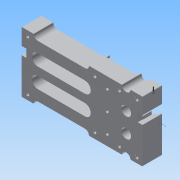
# Autodesk Inventor part: Core_bottom-im
Saved by Autodesk Inventor 2016 (Build 200138000, 138)
## iProperties
Created: 2015-05-18
Part Number: Core_bottom-im
Material: ABS Plastic
Document SubType Name: Modeling
Designer: Openlab
Density: 1.06 g/cm^3
Appearance: Smooth - White
Mass: 36.0444 g
Surface Area: 283.752 cm^2
Volume: 34.0041 cm^3
Author: Openlab
Autodesk Inventor part; units mm, degrees
ref_plane "YZ Plane" through (0, 0, 0) normal (1, 0, 0) x (0, 1, 0)
ref_plane "XZ Plane" through (0, 0, 0) normal (0, 1, 0) x (-1, 0, 0)
ref_plane "XY Plane" through (0, 0, 0) normal (0, 0, 1) x (1, 0, 0)
sketch "Sketch1" plane through (0, 0, 0) normal (0, 1, 0) x (-1, 0, 0)
  line L0 (6.75, 23.75) -> (-6.75, 23.75)
  line L1 (-6.75, 23.75) -> (-6.75, 19.5)
  line L2 (-6.75, 10.25) -> (6.75, 10.25)
  line L3 (6.75, 10.25) -> (6.75, 14.5)
  line L4 (56.9183, 17) -> (21.35, 17) construction
  line L5 (69.8, -24.75) -> (69.8, -20.1)
  line L6 (-26.8, 24.75) -> (-26.8, 12.5)
  line L7 (9.25, 15) -> (7.25, 15)
  line L8 (7.25, 19) -> (9.25, 19)
  line L9 (-7.25, 15) -> (-9.25, 15)
  line L10 (-9.25, 19) -> (-7.25, 19)
  line L11 (-12.05, 19) -> (-24.5, 19)
  line L12 (-12.05, 15) -> (-24.5, 15)
  line L13 (21.8266, 8.5) -> (74, 8.5) construction
  line L14 (67.5, 20.5) -> (66, 20.5)
  line L15 (66, 13.5) -> (67.5, 13.5)
  line L16 (-31, 4.5) -> (-31, -25.75)
  line L17 (21.35, -8.5) -> (74, -8.5) construction
  line L18 (6.75, 6.75) -> (-6.75, 6.75)
  line L19 (-6.75, 6.75) -> (-6.75, 2.5)
  line L20 (-6.75, -6.75) -> (6.75, -6.75)
  line L21 (6.75, -6.75) -> (6.75, -2.5)
  line L22 (56.8064, 0) -> (19.3437, 0) construction
  line L23 (0, 20.1335) -> (0, -26.25) construction
  line L24 (9.25, -2) -> (7.25, -2)
  line L25 (7.25, 2) -> (9.25, 2)
  line L26 (67.5, 3.5) -> (66, 3.5)
  line L27 (66, -3.5) -> (67.5, -3.5)
  line L28 (6.75, -10.25) -> (-6.75, -10.25)
  line L29 (6.75, -23.75) -> (6.75, -19.5)
  line L30 (-6.75, -23.75) -> (6.75, -23.75)
  line L31 (55.9522, -17) -> (21.0014, -17) construction
  line L32 (67.5, -13.5) -> (66, -13.5)
  line L33 (66, -20.5) -> (67.5, -20.5)
  line L34 (9.25, -19) -> (7.25, -19)
  line L35 (73.5, 5) -> (72.5, 5)
  line L36 (70.3, 12) -> (72.5, 12)
  line L37 (-9.25, -15) -> (-7.25, -15)
  line L38 (-7.25, -19) -> (-9.25, -19)
  line L39 (-12.05, -19) -> (-24.5, -19)
  line L40 (-9.25, 2) -> (-7.25, 2)
  line L41 (-7.25, -2) -> (-9.25, -2)
  line L42 (-12.05, -2) -> (-24.5, -2)
  line L43 (-29.5, 5) -> (-30.5, 5)
  line L44 (-30.5, 12) -> (-29.5, 12)
  line L45 (67.5, 5.5) -> (66, 5.5)
  line L46 (66, 5.5) -> (66, 11.5)
  line L47 (66, 11.5) -> (67.5, 11.5)
  line L48 (-24.5, 5.5) -> (-23, 5.5)
  line L49 (-23, 5.5) -> (-23, 11.5)
  line L50 (-23, 11.5) -> (-24.5, 11.5)
  line L51 (-25, 24.75) -> (-25, 19.5)
  line L52 (-25, 5) -> (-25, 2.5)
  arc A0 (18.9998, 13.5) -> (19, 3.5) centre (19, 8.5) ccw
  arc A1 (60, 3.5) -> (60, 13.5) centre (60, 8.5) ccw
  arc A2 (19, -3.5) -> (19, -13.5) centre (19, -8.5) ccw
  arc A3 (60, -13.5) -> (60, -3.5) centre (60, -8.5) ccw
  line L53 (18.9998, 13.5) -> (60, 13.5)
  line L54 (19, 3.5) -> (60, 3.5)
  line L55 (19, -3.5) -> (60, -3.5)
  line L56 (19, -13.5) -> (60, -13.5)
  arc A4 (-16.55, -12.5) -> (-16.55, -4.5) centre (-16.55, -8.5) ccw
  line L57 (72.5, -24.75) -> (72.5, -19.6)
  line L58 (-29.5, 24.75) -> (-29.5, 12)
  arc A5 (-17, -4.5) -> (-17, -12.5) centre (-17, -8.5) ccw
  arc A6 (-17, 12.5) -> (-17, 4.5) centre (-17, 8.5) ccw
  line L59 (-16.55, -12.5) -> (-17, -12.5)
  line L60 (-17, -4.5) -> (-16.55, -4.5)
  line L61 (-17, 4.5) -> (-16.55, 4.5)
  line L62 (-16.55, 12.5) -> (-17, 12.5)
  arc A7 (-16.55, 4.5) -> (-16.55, 12.5) centre (-16.55, 8.5) ccw
  line L63 (59.3387, -15) -> (12.05, -15)
  line L64 (59.3387, -19) -> (12.05, -19)
  line L65 (59.3387, -2) -> (12.05, -2)
  line L66 (59.3387, 2) -> (12.05, 2)
  line L67 (59.3387, 15) -> (12.05, 15)
  line L68 (59.3387, 19) -> (12.05, 19)
  arc A8 (61, -14.4) -> (59.3387, -15) centre (61, -17) ccw
  arc A9 (59.3387, -19) -> (61, -19.6) centre (61, -17) ccw
  arc A10 (61, 2.6) -> (59.3387, 2) centre (61, 0) ccw
  arc A11 (59.3387, -2) -> (61, -2.6) centre (61, 0) ccw
  arc A12 (61, 19.6) -> (59.3387, 19) centre (61, 17) ccw
  arc A13 (59.3387, 15) -> (61, 14.4) centre (61, 17) ccw
  arc A14 (63.4725, -25.8125) -> (60, -22.75) centre (60, -26.25) ccw
  arc A15 (19, -22.75) -> (15.5275, -25.8125) centre (19, -26.25) ccw
  arc A16 (64.7697, -24.75) -> (60, -21.25) centre (60, -26.25) ccw
  line L69 (60, -21.25) -> (18.9998, -21.25)
  line L70 (63.9686, -26.25) -> (73.5, -26.25)
  line L71 (60, -22.75) -> (19, -22.75)
  arc A17 (18.9998, -21.25) -> (14.2303, -24.75) centre (19, -26.25) ccw
  arc A18 (14.2559, 24.6709) -> (18.9998, 21.25) centre (19, 26.25) ccw
  arc A19 (15.5275, 25.8125) -> (19, 22.75) centre (19, 26.25) ccw
  line L72 (60, 22.75) -> (19, 22.75)
  line L73 (60, 21.25) -> (18.9998, 21.25)
  line L74 (64.7697, 24.75) -> (69.8, 24.75)
  line L75 (73.5, 26.25) -> (63.9686, 26.25)
  arc A20 (60, 22.75) -> (63.4725, 25.8125) centre (60, 26.25) ccw
  arc A21 (60, 21.25) -> (64.7697, 24.75) centre (60, 26.25) ccw
  arc A22 (-13.0775, -25.8125) -> (-16.55, -22.75) centre (-16.55, -26.25) ccw
  arc A23 (-17, -22.75) -> (-20.4725, -25.8125) centre (-17, -26.25) ccw
  line L76 (-16.55, -21.25) -> (-17, -21.25)
  line L77 (-16.55, -22.75) -> (-17, -22.75)
  arc A24 (-17, -21.25) -> (-21.7697, -24.75) centre (-17, -26.25) ccw
  arc A25 (-11.7803, -24.75) -> (-16.55, -21.25) centre (-16.55, -26.25) ccw
  line L78 (14.2303, -24.75) -> (-11.7803, -24.75)
  line L79 (-21.7697, -24.75) -> (-29.5, -24.75)
  line L80 (-30.5, -26.25) -> (-20.9686, -26.25)
  line L81 (14.7303, -26.25) -> (15.0314, -26.25)
  line L82 (-16.55, 21.25) -> (-17, 21.25)
  line L83 (-16.55, 22.75) -> (-17, 22.75)
  arc A26 (-20.4725, 25.8125) -> (-17, 22.75) centre (-17, 26.25) ccw
  arc A27 (-16.55, 22.75) -> (-13.0775, 25.8125) centre (-16.55, 26.25) ccw
  arc A28 (-21.7697, 24.75) -> (-17, 21.25) centre (-17, 26.25) ccw
  arc A29 (-16.55, 21.25) -> (-11.836, 24.5833) centre (-16.55, 26.25) ccw
  line L84 (15.0314, 26.25) -> (14.7303, 26.25)
  line L85 (-20.9686, 26.25) -> (-30.5, 26.25)
  line L86 (-29.5, 24.75) -> (-21.7697, 24.75)
  line L87 (-11.8074, 24.75) -> (14.2303, 24.75)
  line L88 (14.2303, -24.75) -> (14.2303, -25.75)
  line L89 (-11.7803, -24.75) -> (-11.7803, -25.75)
  line L90 (-11.8074, 24.75) -> (-11.8074, 25.75)
  line L91 (14.2303, 24.8288) -> (14.2303, 25.75)
  line L92 (72.5, 12) -> (73.5, 12)
  line L93 (72.5, 5) -> (70.3, 5)
  line L94 (-27.3, 12) -> (-29.5, 12)
  line L95 (-27.3, 5) -> (-29.5, 5)
  line L96 (11.55, -21) -> (9.75, -21)
  line L97 (9.75, 21) -> (11.55, 21)
  line L98 (-9.75, -21) -> (-11.55, -21)
  line L99 (-11.55, 21) -> (-9.75, 21)
  line L100 (11.55, -2.5) -> (11.55, -14.5)
  line L101 (11.55, -19.5) -> (11.55, -21)
  line L102 (9.75, -21) -> (9.75, -19.5)
  line L103 (11.55, 21) -> (11.55, 19.5)
  line L104 (11.55, 14.5) -> (11.55, 2.5)
  line L105 (9.75, 2.5) -> (9.75, 14.5)
  line L106 (9.75, 19.5) -> (9.75, 21)
  line L107 (-9.75, -2.5) -> (-9.75, -14.5)
  line L108 (-9.75, -19.5) -> (-9.75, -21)
  line L109 (-11.55, -21) -> (-11.55, -19.5)
  line L110 (-11.55, -14.5) -> (-11.55, -2.5)
  line L111 (-9.75, 21) -> (-9.75, 19.5)
  line L112 (-9.75, 14.5) -> (-9.75, 2.5)
  line L113 (-11.55, 2.5) -> (-11.55, 14.5)
  line L114 (-11.55, 19.5) -> (-11.55, 21)
  line L115 (67.5, -11.5) -> (66, -11.5)
  line L116 (66, -11.5) -> (66, -5.5)
  line L117 (66, -5.5) -> (67.5, -5.5)
  line L118 (68, -21) -> (68, -24.75)
  arc A30 (9.75, -19.5) -> (9.25, -19) centre (9.25, -19.5) ccw
  arc A31 (12.05, -19) -> (11.55, -19.5) centre (12.05, -19.5) ccw
  arc A32 (9.75, -2.5) -> (9.25, -2) centre (9.25, -2.5) ccw
  arc A33 (12.05, -2) -> (11.55, -2.5) centre (12.05, -2.5) ccw
  arc A34 (11.55, 2.5) -> (12.05, 2) centre (12.05, 2.5) ccw
  arc A35 (9.25, 2) -> (9.75, 2.5) centre (9.25, 2.5) ccw
  arc A36 (9.75, 14.5) -> (9.25, 15) centre (9.25, 14.5) ccw
  arc A37 (12.05, 15) -> (11.55, 14.5) centre (12.05, 14.5) ccw
  arc A38 (11.55, 19.5) -> (12.05, 19) centre (12.05, 19.5) ccw
  arc A39 (9.25, 19) -> (9.75, 19.5) centre (9.25, 19.5) ccw
  arc A40 (-9.75, 19.5) -> (-9.25, 19) centre (-9.25, 19.5) ccw
  arc A41 (-12.05, 19) -> (-11.55, 19.5) centre (-12.05, 19.5) ccw
  arc A42 (-11.55, 14.5) -> (-12.05, 15) centre (-12.05, 14.5) ccw
  arc A43 (-9.25, 15) -> (-9.75, 14.5) centre (-9.25, 14.5) ccw
  arc A44 (-9.75, 2.5) -> (-9.25, 2) centre (-9.25, 2.5) ccw
  arc A45 (-12.05, 2) -> (-11.55, 2.5) centre (-12.05, 2.5) ccw
  arc A46 (-11.55, -2.5) -> (-12.05, -2) centre (-12.05, -2.5) ccw
  arc A47 (-9.25, -2) -> (-9.75, -2.5) centre (-9.25, -2.5) ccw
  arc A48 (-9.75, -14.5) -> (-9.25, -15) centre (-9.25, -14.5) ccw
  arc A49 (-12.05, -15) -> (-11.55, -14.5) centre (-12.05, -14.5) ccw
  arc A50 (-9.25, -19) -> (-9.75, -19.5) centre (-9.25, -19.5) ccw
  arc A51 (-11.55, -19.5) -> (-12.05, -19) centre (-12.05, -19.5) ccw
  line L119 (65.5, -19.6) -> (61, -19.6)
  line L120 (66, -13.5) -> (66, -13.9)
  line L121 (61, -14.4) -> (65.5, -14.4)
  line L122 (65.5, -2.6) -> (61, -2.6)
  line L123 (66, 3.5) -> (66, 3.1)
  line L124 (66, -3.1) -> (66, -3.5)
  line L125 (61, 2.6) -> (65.5, 2.6)
  line L126 (65.5, 14.4) -> (61, 14.4)
  line L127 (66, 20.5) -> (66, 20.1)
  line L128 (66, 13.9) -> (66, 13.5)
  line L129 (61, 19.6) -> (65.5, 19.6)
  arc A52 (65.5, -14.4) -> (66, -13.9) centre (65.5, -13.9) ccw
  arc A53 (68, -12) -> (67.5, -11.5) centre (67.5, -12) ccw
  arc A54 (67.5, -5.5) -> (68, -5) centre (67.5, -5) ccw
  arc A55 (68, 5) -> (67.5, 5.5) centre (67.5, 5) ccw
  arc A56 (67.5, 11.5) -> (68, 12) centre (67.5, 12) ccw
  arc A57 (66, -3.1) -> (65.5, -2.6) centre (65.5, -3.1) ccw
  arc A58 (65.5, 2.6) -> (66, 3.1) centre (65.5, 3.1) ccw
  arc A59 (66, 13.9) -> (65.5, 14.4) centre (65.5, 13.9) ccw
  arc A60 (65.5, 19.6) -> (66, 20.1) centre (65.5, 20.1) ccw
  line L130 (72.5, -2.6) -> (72.5, 2.6)
  line L131 (72.5, -2.6) -> (70.3, -2.6)
  line L132 (66, -20.5) -> (66, -20.1)
  arc A61 (66, -20.1) -> (65.5, -19.6) centre (65.5, -20.1) ccw
  line L133 (68, -13) -> (68, -12)
  line L134 (68, 4) -> (68, 5)
  line L135 (68, 21) -> (68, 24.75)
  line L136 (72.5, -19.6) -> (72.5, -14.4)
  line L137 (72.5, -19.6) -> (70.3, -19.6)
  line L138 (72.5, -24.75) -> (69.8, -24.75)
  line L139 (69.8, -24.75) -> (68, -24.75)
  line L140 (68, -24.75) -> (64.7697, -24.75)
  line L141 (70.3, -14.4) -> (72.5, -14.4)
  line L142 (72.5, -14.4) -> (72.5, -2.6)
  line L143 (69.8, -13.9) -> (69.8, -3.1)
  line L144 (68, -4) -> (68, -5)
  line L145 (72.5, 2.6) -> (72.5, 5)
  line L146 (70.3, 2.6) -> (72.5, 2.6)
  line L147 (69.8, 3.1) -> (69.8, 4.5)
  line L148 (72.5, 14.4) -> (72.5, 19.6)
  line L149 (72.5, 14.4) -> (70.3, 14.4)
  line L150 (74, -25.75) -> (74, 4.5)
  line L151 (72.5, 19.6) -> (72.5, 24.75)
  line L152 (69.8, 20.1) -> (69.8, 24.75)
  line L153 (70.3, 19.6) -> (72.5, 19.6)
  line L154 (72.5, 12) -> (72.5, 14.4)
  line L155 (69.8, 24.75) -> (72.5, 24.75)
  line L156 (69.8, 12.5) -> (69.8, 13.9)
  line L157 (68, 13) -> (68, 12)
  arc A62 (67.5, -13.5) -> (68, -13) centre (67.5, -13) ccw
  arc A63 (68, -4) -> (67.5, -3.5) centre (67.5, -4) ccw
  arc A64 (67.5, 3.5) -> (68, 4) centre (67.5, 4) ccw
  arc A65 (68, 13) -> (67.5, 13.5) centre (67.5, 13) ccw
  arc A66 (67.5, 20.5) -> (68, 21) centre (67.5, 21) ccw
  arc A67 (70.3, -19.6) -> (69.8, -20.1) centre (70.3, -20.1) ccw
  arc A68 (69.8, -13.9) -> (70.3, -14.4) centre (70.3, -13.9) ccw
  arc A69 (70.3, -2.6) -> (69.8, -3.1) centre (70.3, -3.1) ccw
  arc A70 (69.8, 3.1) -> (70.3, 2.6) centre (70.3, 3.1) ccw
  arc A71 (70.3, 14.4) -> (69.8, 13.9) centre (70.3, 13.9) ccw
  arc A72 (69.8, 20.1) -> (70.3, 19.6) centre (70.3, 20.1) ccw
  line L158 (69.8, 5) -> (69.8, 12)
  line L159 (-25, 14.5) -> (-25, 12)
  line L160 (-25, -2.5) -> (-25, -14.5)
  line L161 (-25, -19.5) -> (-25, -24.75)
  line L162 (-29.5, 5) -> (-29.5, -24.75)
  arc A73 (-25, 12) -> (-24.5, 11.5) centre (-24.5, 12) ccw
  arc A74 (-24.5, 5.5) -> (-25, 5) centre (-24.5, 5) ccw
  arc A75 (68, -21) -> (67.5, -20.5) centre (67.5, -21) ccw
  arc A76 (70.3, 5) -> (69.8, 4.5) centre (70.3, 4.5) ccw
  arc A77 (69.8, 12.5) -> (70.3, 12) centre (70.3, 12.5) ccw
  line L163 (69.8, 5) -> (70.3, 5)
  line L164 (69.8, 12) -> (70.3, 12)
  arc A78 (74, 4.5) -> (73.5, 5) centre (73.5, 4.5) ccw
  line L165 (74, 25.75) -> (74, 12.5)
  arc A79 (73.5, 12) -> (74, 12.5) centre (73.5, 12.5) ccw
  line L166 (74, 4.5) -> (74, 12.5)
  arc A80 (-30.5, 5) -> (-31, 4.5) centre (-30.5, 4.5) ccw
  line L167 (-31, 12.5) -> (-31, 25.75)
  arc A81 (-31, 12.5) -> (-30.5, 12) centre (-30.5, 12.5) ccw
  line L168 (-31, 4.5) -> (-31, 12.5)
  line L169 (-26.8, -24.75) -> (-26.8, 4.5)
  arc A82 (-27.3, 12) -> (-26.8, 12.5) centre (-27.3, 12.5) ccw
  arc A83 (-26.8, 4.5) -> (-27.3, 5) centre (-27.3, 4.5) ccw
  line L170 (-26.8, 5) -> (-26.8, 12)
  line L171 (-27.3, 12) -> (-26.8, 12)
  line L172 (-27.3, 5) -> (-26.8, 5)
  arc A84 (73.5, -26.25) -> (74, -25.75) centre (73.5, -25.75) ccw
  arc A85 (63.4725, -25.8125) -> (63.9686, -26.25) centre (63.9686, -25.75) ccw
  arc A86 (15.0314, -26.25) -> (15.5275, -25.8125) centre (15.0314, -25.75) ccw
  arc A87 (-13.0775, -25.8125) -> (-12.5814, -26.25) centre (-12.5814, -25.75) ccw
  arc A88 (-20.9686, -26.25) -> (-20.4725, -25.8125) centre (-20.9686, -25.75) ccw
  arc A89 (-31, -25.75) -> (-30.5, -26.25) centre (-30.5, -25.75) ccw
  arc A90 (-30.5, 26.25) -> (-31, 25.75) centre (-30.5, 25.75) ccw
  arc A91 (-20.4725, 25.8125) -> (-20.9686, 26.25) centre (-20.9686, 25.75) ccw
  arc A92 (-12.5814, 26.25) -> (-13.0775, 25.8125) centre (-12.5814, 25.75) ccw
  arc A93 (15.5275, 25.8125) -> (15.0314, 26.25) centre (15.0314, 25.75) ccw
  arc A94 (63.9686, 26.25) -> (63.4725, 25.8125) centre (63.9686, 25.75) ccw
  arc A95 (74, 25.75) -> (73.5, 26.25) centre (73.5, 25.75) ccw
  line L173 (6.75, -19.5) -> (6.75, -14.5)
  line L174 (6.75, -14.5) -> (6.75, -10.25)
  line L175 (-6.75, -14.5) -> (-6.75, -19.5)
  line L176 (-6.75, -19.5) -> (-6.75, -23.75)
  arc A96 (7.25, -19) -> (6.75, -19.5) centre (7.25, -19.5) ccw
  arc A97 (6.75, -14.5) -> (7.25, -15) centre (7.25, -14.5) ccw
  arc A98 (-6.75, -19.5) -> (-7.25, -19) centre (-7.25, -19.5) ccw
  arc A99 (11.55, -14.5) -> (12.05, -15) centre (12.05, -14.5) ccw
  line L177 (9.75, -2.5) -> (9.75, -14.5)
  line L178 (9.25, -15) -> (7.25, -15)
  arc A100 (9.25, -15) -> (9.75, -14.5) centre (9.25, -14.5) ccw
  line L179 (-6.75, -10.25) -> (-6.75, -14.5)
  arc A101 (-7.25, -15) -> (-6.75, -14.5) centre (-7.25, -14.5) ccw
  line L180 (6.75, -2.5) -> (6.75, 2.5)
  line L181 (6.75, 2.5) -> (6.75, 6.75)
  line L182 (-6.75, -2.5) -> (-6.75, -6.75)
  line L183 (-6.75, 2.5) -> (-6.75, -2.5)
  line L184 (6.75, 14.5) -> (6.75, 19.5)
  line L185 (6.75, 19.5) -> (6.75, 23.75)
  line L186 (-6.75, 19.5) -> (-6.75, 14.5)
  line L187 (-6.75, 14.5) -> (-6.75, 10.25)
  arc A102 (7.25, -2) -> (6.75, -2.5) centre (7.25, -2.5) ccw
  arc A103 (6.75, 2.5) -> (7.25, 2) centre (7.25, 2.5) ccw
  arc A104 (-6.75, -2.5) -> (-7.25, -2) centre (-7.25, -2.5) ccw
  arc A105 (-7.25, 2) -> (-6.75, 2.5) centre (-7.25, 2.5) ccw
  arc A106 (7.25, 15) -> (6.75, 14.5) centre (7.25, 14.5) ccw
  arc A107 (6.75, 19.5) -> (7.25, 19) centre (7.25, 19.5) ccw
  arc A108 (-7.25, 19) -> (-6.75, 19.5) centre (-7.25, 19.5) ccw
  arc A109 (-6.75, 14.5) -> (-7.25, 15) centre (-7.25, 14.5) ccw
  arc A110 (14.2303, -25.75) -> (14.7303, -26.25) centre (14.7303, -25.75) ccw
  line L188 (-12.5814, -26.25) -> (-12.2803, -26.25)
  line L189 (-12.2803, -26.25) -> (14.7303, -26.25)
  arc A111 (-12.2803, -26.25) -> (-11.7803, -25.75) centre (-12.2803, -25.75) ccw
  arc A112 (14.7303, 26.25) -> (14.2303, 25.75) centre (14.7303, 25.75) ccw
  line L190 (-12.5814, 26.25) -> (-12.3074, 26.25)
  line L191 (-12.3074, 26.25) -> (14.7303, 26.25)
  arc A113 (-11.8074, 25.75) -> (-12.3074, 26.25) centre (-12.3074, 25.75) ccw
  arc A114 (14.2303, 24.8288) -> (14.2559, 24.6709) centre (14.7303, 24.8288) ccw
  arc A115 (-11.836, 24.5833) -> (-11.8074, 24.75) centre (-12.3074, 24.75) ccw
  line L192 (-24.5, 2) -> (-12.05, 2)
  line L193 (-24.5, -15) -> (-12.05, -15)
  arc A116 (-24.5, -19) -> (-25, -19.5) centre (-24.5, -19.5) ccw
  arc A117 (-25, -14.5) -> (-24.5, -15) centre (-24.5, -14.5) ccw
  arc A118 (-24.5, -2) -> (-25, -2.5) centre (-24.5, -2.5) ccw
  arc A119 (-25, 2.5) -> (-24.5, 2) centre (-24.5, 2.5) ccw
  arc A120 (-24.5, 15) -> (-25, 14.5) centre (-24.5, 14.5) ccw
  arc A121 (-25, 19.5) -> (-24.5, 19) centre (-24.5, 19.5) ccw
  point P0 (0, 0)
  point P1 (0, -17)
  point P2 (0, 0)
  point P3 (0, 17)
  point P4 (72.5, -8.5)
  dimension "d125" = 7
  dimension "d159" = 6
  dimension "d164" = 6
  dimension "d286" = 5
  dimension "d287" = 1.5
  dimension "d292" = 1.5
  dimension "d298" = 1.5
  dimension "d314" = 2.7
  dimension "d324" = 2.7
  dimension "d344" = 7
  dimension "d374" = 25
  dimension "d379" = 5
  dimension "d381" = 1.8
  dimension "d390" = 13.5
  dimension "d392" = 8
  dimension "d406" = 7
  dimension "d407" = 7
  dimension "d421" = 2
  dimension "d436" = 1.8
  dimension "d437" = 8
  dimension "d440" = 1.5
  dimension "d443" = 4
  dimension "d445" = 0.5
  dimension "d446" = 68
  dimension "d447" = 5.2
  dimension "d448" = 7
  dimension "d449" = 5.2
  dimension "d450" = 5.2
  dimension "d452" = 2
  dimension "d453" = 1.5
  dimension "d454" = 0.5
  dimension "d455" = 0.5
  dimension "d456" = 0.5
  dimension "d462" = 7
  dimension "d463" = 0.5
  dimension "d470" = 3
  dimension "d471" = 3
  dimension "d476" = 0.5
  dimension "d477" = 0.5
  dimension "d485" = 17
  dimension "d486" = 49.5
  dimension "d488" = 4
  dimension "d489" = 4
  dimension "d512" = 13.5
  dimension "d513" = 13.5
  dimension "d514" = 13.5
  dimension "d515" = 19
  dimension "d525" = 2.7
  dimension "d526" = 1.8
  dimension "d527" = 102
  dimension "d528" = 4
  dimension "d529" = 4
  dimension "d534" = 16.55
  constraints: 390 end point, 247 point on circle, 225 tangent, 155 perpendicular, 122 centre point, 108 equal radius, 101 collinear, 55 parallel, 31 point on line, 25 horizontal, 14 vertical alignment, 9 coincident, 9 vertical, 7 horizontal alignment, 1 midpoint, 34 other
  measures "d125" distance of L14.end L15.start
  measures "d159" distance of L45.end L46.end
  measures "d164" distance of L48.end L49.end
  measures "d286" radius of A16
  measures "d287" radial gap between concentric circles of A14 A16
  measures "d292" distance between parallel lines of L75 L74
  measures "d298" distance between parallel lines of L79 L80
  measures "d314" distance between parallel lines of L58 L6
  measures "d324" distance between parallel lines of L5 L57
  measures "d344" distance between parallel lines of L93 L36
  measures "d374" distance between parallel lines of L51 L23
  measures "d379" radius of A2
  measures "d381" distance of L96.start L96.end
  measures "d390" distance between parallel lines of L0 L2
  measures "d392" distance from line of A14.centre L118
  measures "d406" distance between parallel lines of L26 L27
  measures "d407" distance between parallel lines of L32 L33
  measures "d421" distance between parallel lines of L46 L134
  measures "d436" distance between parallel lines of L118 L5
  measures "d437" distance from line of L161 A24.centre
  measures "d440" distance between parallel lines of L16 L162
  measures "d443" distance between parallel lines of L11 L12
  measures "d445" radius of A32
  measures "d446" distance between parallel lines of L135 L23
  measures "d447" distance between parallel lines of L141 L137
  measures "d448" distance from line of A10.centre L144
  measures "d449" distance between parallel lines of L146 L131
  measures "d450" distance between parallel lines of L153 L149
  measures "d452" distance between parallel lines of L52 L49
  measures "d453" distance between parallel lines of L57 L150
  measures "d454" radius of A76
  measures "d455" radius of A78
  measures "d456" radius of A79
  measures "d462" distance between parallel lines of L44 L43
  measures "d463" radius of A84
  measures "d470" distance between parallel lines of L29 L102
  measures "d471" distance between parallel lines of L108 L176
  measures "d476" radius of A110
  measures "d477" radius of A111
  measures "d485" distance between parallel lines of L22 L31
  measures "d486" distance between parallel lines of L138 L155
  measures "d488" distance between parallel lines of L192 L42
  measures "d489" distance between parallel lines of L193 L39
  measures "d512" distance between parallel lines of L20 L18
  measures "d513" distance between parallel lines of L30 L28
  measures "d514" distance between parallel lines of L187 L3
  measures "d515" distance from line of L23 A15.centre
  measures "d525" distance of L79.end L169.start
  measures "d526" distance between parallel lines of L169 L161
  measures "d527" distance between parallel lines of L58 L151
  measures "d528" distance between parallel lines of L4 L97
  measures "d529" radius of A5
  measures "d534" distance from line of A25.centre L23
extrude "Extrusion33" add sketch "Sketch1" against normal blind 1.5 contours L185 L184 L3 L2 L187 L186 L1 L0 | L0 L1 A108 L10 A40 L111 L99 L114 A41 L11 A121 L51 L86 A28 L82 A29 A115 L90 A113 L191 A112 L91 A114 A18 L73 A21 L74 L135 A66 L14 L127 A60 L129 A12 L68 A38 L103 L97 L106 A39 L8 A107 L185 | A107 L8 A39 L106 L97 L103 A38 L68 A12 L129 A60 L127 L14 A66 L135 L74 L152 A72 L153 L148 L149 A71 L156 A77 L164 L158 L163 A76 L147 A70 L146 L130 L131 A69 L143 A68 L141 L136 L137 A67 L5 L139 L118 A75 L33 L132 A61 L119 A9 L64 A31 L101 L96 L102 A30 L34 A96 L173 A97 L178 A100 L177 A32 L24 A102 L180 A103 L25 A35 L105 A36 L7 A106 L184 | L186 A109 L9 A43 L112 A44 L40 A105 L183 A104 L41 A47 L107 A48 L37 A101 L175 A98 L38 A50 L108 L98 L109 A51 L39 A116 L161 L79 L169 A83 L172 L170 L171 A82 L6 L86 L51 A121 L11 A41 L114 L99 L111 A40 L10 A108 | A106 L7 A36 L105 A35 L25 A103 L181 L18 L19 A105 L40 A44 L112 A43 L9 A109 L187 L2 L3 | L180 L21 L20 L182 L183 L19 L18 L181 | A102 L24 A32 L177 A100 L178 A97 L174 L28 L179 A101 L37 A48 L107 A47 L41 A104 L182 L20 L21 | L86 L58 L44 A81 L167 A90 L85 A91 A26 L83 A27 A92 L190 A113 L90 A115 A29 L82 A28 | L6 A82 L94 L58 L86 | L74 A21 L73 A18 A114 L91 A112 L84 A93 A19 L72 A20 A94 L75 A95 L165 A79 L92 L154 L148 L151 L155 | L173 L29 L30 L176 L175 L179 L28 L174 | L155 L151 L153 A72 L152 | A83 L169 L79 L162 L95 | A80 L43 L162 L79 A24 L76 A25 L89 A111 L188 A87 A22 L77 A23 A88 L80 A89 L16 | A96 L34 A30 L102 L96 L101 A31 L64 A9 L119 A61 L132 L33 A75 L118 L140 A16 L69 A17 L78 A25 L76 A24 L79 L161 A116 L39 A51 L109 L98 L108 A50 L38 A98 L176 L30 L29 | L154 L36 A77 L156 A71 L149 | L150 A84 L70 A85 A14 L71 A15 A86 L81 A110 L88 A17 L69 A16 L140 L139 L138 L57 L136 L142 L130 L145 L35 A78 | L78 L88 A110 L189 A111 L89 | L93 L145 L146 A70 L147 A76 | L142 L141 A68 L143 A69 L131 | L57 L138 L5 A67 L137 | A42 L113 A45 L192 A119 L52 A74 L48 L49 L50 A73 L159 A120 L12 | L15 A65 L157 A56 L47 L46 L45 A55 L134 A64 L26 L123 A58 L125 A10 L66 A34 L104 A37 L67 A13 L126 A59 L128 | L27 A63 L144 A54 L117 L116 L115 A53 L133 A62 L32 L120 A52 L121 A8 L63 A99 L100 A33 L65 A11 L122 A57 L124 | A46 L110 A49 L193 A117 L160 A118 L42
hole "Hole3" at (0, 0, -17) at (0, 0, 0) at (0, 0, 17) direction (0, -1, 0) diameter 3 end through all countersink diameter 6 countersink angle 120
extrude "Extrusion30" add sketch "Sketch1" along normal blind 12.5 contours L0 L1 A108 L10 A40 L111 L99 L114 A41 L11 A121 L51 L86 A28 L82 A29 A115 L90 A113 L191 A112 L91 A114 A18 L73 A21 L74 L135 A66 L14 L127 A60 L129 A12 L68 A38 L103 L97 L106 A39 L8 A107 L185 | A106 L7 A36 L105 A35 L25 A103 L181 L18 L19 A105 L40 A44 L112 A43 L9 A109 L187 L2 L3 | A102 L24 A32 L177 A100 L178 A97 L174 L28 L179 A101 L37 A48 L107 A47 L41 A104 L182 L20 L21 | L6 A82 L94 L58 L86 | L155 L151 L153 A72 L152 | A83 L169 L79 L162 L95 | A96 L34 A30 L102 L96 L101 A31 L64 A9 L119 A61 L132 L33 A75 L118 L140 A16 L69 A17 L78 A25 L76 A24 L79 L161 A116 L39 A51 L109 L98 L108 A50 L38 A98 L176 L30 L29 | L154 L36 A77 L156 A71 L149 | L78 L88 A110 L189 A111 L89 | L93 L145 L146 A70 L147 A76 | L142 L141 A68 L143 A69 L131 | L57 L138 L5 A67 L137 | A42 L113 A45 L192 A119 L52 A74 L48 L49 L50 A73 L159 A120 L12 | L15 A65 L157 A56 L47 L46 L45 A55 L134 A64 L26 L123 A58 L125 A10 L66 A34 L104 A37 L67 A13 L126 A59 L128 | L27 A63 L144 A54 L117 L116 L115 A53 L133 A62 L32 L120 A52 L121 A8 L63 A99 L100 A33 L65 A11 L122 A57 L124 | A46 L110 A49 L193 A117 L160 A118 L42
extrude "Extrusion29" add sketch "Sketch1" along normal blind 15.5 contours L86 L58 L44 A81 L167 A90 L85 A91 A26 L83 A27 A92 L190 A113 L90 A115 A29 L82 A28 | L74 A21 L73 A18 A114 L91 A112 L84 A93 A19 L72 A20 A94 L75 A95 L165 A79 L92 L154 L148 L151 L155 | A80 L43 L162 L79 A24 L76 A25 L89 A111 L188 A87 A22 L77 A23 A88 L80 A89 L16 | L150 A84 L70 A85 A14 L71 A15 A86 L81 A110 L88 A17 L69 A16 L140 L139 L138 L57 L136 L142 L130 L145 L35 A78
extrude "Extrusion32" add sketch "Sketch1" along normal blind 2.5 contours A107 L8 A39 L106 L97 L103 A38 L68 A12 L129 A60 L127 L14 A66 L135 L74 L152 A72 L153 L148 L149 A71 L156 A77 L164 L158 L163 A76 L147 A70 L146 L130 L131 A69 L143 A68 L141 L136 L137 A67 L5 L139 L118 A75 L33 L132 A61 L119 A9 L64 A31 L101 L96 L102 A30 L34 A96 L173 A97 L178 A100 L177 A32 L24 A102 L180 A103 L25 A35 L105 A36 L7 A106 L184 | L186 A109 L9 A43 L112 A44 L40 A105 L183 A104 L41 A47 L107 A48 L37 A101 L175 A98 L38 A50 L108 L98 L109 A51 L39 A116 L161 L79 L169 A83 L172 L170 L171 A82 L6 L86 L51 A121 L11 A41 L114 L99 L111 A40 L10 A108 | L154 L36 A77 L156 A71 L149 | A42 L113 A45 L192 A119 L52 A74 L48 L49 L50 A73 L159 A120 L12 | L15 A65 L157 A56 L47 L46 L45 A55 L134 A64 L26 L123 A58 L125 A10 L66 A34 L104 A37 L67 A13 L126 A59 L128 | L27 A63 L144 A54 L117 L116 L115 A53 L133 A62 L32 L120 A52 L121 A8 L63 A99 L100 A33 L65 A11 L122 A57 L124 | A46 L110 A49 L193 A117 L160 A118 L42
sketch "Sketch6" plane through (0, -1.5, 0) normal (0, -1, 0) x (1, 0, 0)
  arc A0 (-73.5, 26.25) -> (-74, 25.75) centre (-73.5, 25.75) ccw projected
  arc A1 (-74, -25.75) -> (-73.5, -26.25) centre (-73.5, -25.75) ccw projected
  arc A2 (30.5, -26.25) -> (31, -25.75) centre (30.5, -25.75) ccw projected
  arc A3 (31, 25.75) -> (30.5, 26.25) centre (30.5, 25.75) ccw projected
  circle A4 centre (-73.5, 25.75) radius 7.5
  circle A5 centre (-73.5, -25.75) radius 7.5
  circle A6 centre (30.5, 25.75) radius 7.5
  circle A7 centre (30.5, -25.75) radius 7.5
  point P0 (0, 0)
  dimension "d497" = 15
  constraints: 4 centre point, 4 coincident, 3 equal radius
  measures "d497" diameter of A4
extrude "Extrusion34" [suppressed]
sketch "Sketch8" plane through (0, 12.5, 0) normal (0, 1, 0) x (1, 0, 0)
  line L0 (26.8, 24.75) -> (26.8, -4.5) projected
  line L1 (25, 19.5) -> (25, 24.75) projected
  line L2 (21.7697, 24.75) -> (29.5, 24.75) projected
  line L3 (26.8, -12.5) -> (26.8, -24.75) projected
  line L4 (29.5, -24.75) -> (21.7697, -24.75) projected
  line L5 (25, -24.75) -> (25, -19.5) projected
  line L6 (-69.8, -24.75) -> (-69.8, -20.1) projected
  line L7 (-64.7697, -24.75) -> (-72.5, -24.75) projected
  line L8 (-68, -21) -> (-68, -24.75) projected
  line L9 (-69.8, 20.1) -> (-69.8, 24.75) projected
  line L10 (-68, 24.75) -> (-68, 21) projected
  line L11 (-72.5, 24.75) -> (-64.7697, 24.75) projected
  line L12 (-69.8, 24.75) -> (-68, 24.75) construction
  line L13 (-68, -21) -> (-68, -24.75) construction
  line L14 (-68, 24.75) -> (-68, 21) construction
  line L15 (26.8, -24.75) -> (25, -24.75) construction
  line L16 (25, 19.5) -> (25, 24.75) construction
  line L17 (25, -24.75) -> (25, -19.5) construction
  line L18 (-68, -24.75) -> (-69.8, -24.75) projected
  line L19 (37.7946, 0) -> (-84.0288, 0) construction
  line L20 (-19, 13.5) -> (-60, 13.5) construction
  line L21 (25, 24.75) -> (26.8, 24.75) construction
  line L22 (-11.55, -21) -> (-11.55, -19.5) projected
  line L23 (-9.75, -19.5) -> (-9.75, -21) projected
  line L24 (-9.75, -21) -> (-11.55, -21) projected
  line L25 (-11.55, 19.5) -> (-11.55, 21) projected
  line L26 (-11.55, 21) -> (-9.75, 21) projected
  line L27 (-9.75, 21) -> (-9.75, 19.5) projected
  line L28 (9.75, 19.5) -> (9.75, 21) projected
  line L29 (9.75, 21) -> (11.55, 21) projected
  line L30 (11.55, 21) -> (11.55, 19.5) projected
  line L31 (9.75, -21) -> (9.75, -19.5) projected
  line L32 (11.55, -21) -> (9.75, -21) projected
  line L33 (11.55, -19.5) -> (11.55, -21) projected
  point P0 (0, 0)
  point P1 (-68.9, 21.75)
  point P2 (-68.9, -21.75)
  point P3 (25.9, -21.75)
  point P4 (25.9, 21.75)
  point P5 (-68.9, -24.75)
  point P6 (-68.9, 24.75)
  point P7 (25.9, -24.75)
  point P8 (25.9, 24.75)
  point P9 (-10.65, 21)
  point P10 (10.65, 21)
  point P11 (-10.65, -21)
  point P12 (10.65, -21)
  dimension "d516" = 3
  constraints: 8 midpoint, 4 vertical alignment, 2 end point, 2 horizontal alignment, 1 parallel, 1 point on line, 1 symmetric about line
  measures "d516" distance from line of point (25.9, -21.75) L4
sketch "Sketch9" plane through (0, -1.5, 0) normal (0, -1, 0) x (1, 0, 0)
  point P0 (0, 0)
  point P1 (25.9, 21.75)
  point P2 (25.9, -21.75)
  point P3 (-68.9, -21.75)
  point P4 (-68.9, 21.75)
  point P5 (-10.65, -21)
  point P6 (10.65, -21)
  point P7 (-10.65, 21)
  point P8 (10.65, 21)
hole "Hole7" at (-68.9, -1.5, -21.75) at (-68.9, -1.5, 21.75) at (25.9, -1.5, 21.75) at (25.9, -1.5, -21.75) at (-10.65, -1.5, -21) at (10.65, -1.5, -21) at (10.65, -1.5, 21) at (-10.65, -1.5, 21) direction (0, 1, 0) diameter 3 depth 8 tip angle 70
sketch "Sketch10" plane through (0, 2.5, 0) normal (0, 1, 0) x (1, 0, 0)
  line L0 (-9.75, -2.5) -> (-9.75, -14.5) projected
  line L1 (-11.55, -14.5) -> (-11.55, -2.5) projected
  line L2 (-9.75, 14.5) -> (-9.75, 2.5) projected
  line L3 (-11.55, 2.5) -> (-11.55, 14.5) projected
  line L4 (9.75, 2.5) -> (9.75, 14.5) projected
  line L5 (11.55, 14.5) -> (11.55, 2.5) projected
  line L6 (11.55, -2.5) -> (11.55, -14.5) projected
  line L7 (9.75, -14.5) -> (9.75, -2.5) projected
  line L8 (11.55, -10.5) -> (9.75, -10.5)
  line L9 (11.55, -6.5) -> (9.75, -6.5)
  line L10 (-9.75, -10.5) -> (-11.55, -10.5)
  line L11 (-9.75, -6.5) -> (-11.55, -6.5)
  line L12 (11.55, 6.5) -> (9.75, 6.5)
  line L13 (11.55, 10.5) -> (9.75, 10.5)
  line L14 (-9.75, 6.5) -> (-11.55, 6.5)
  line L15 (-9.75, 10.5) -> (-11.55, 10.5)
  line L16 (11.55, 0) -> (-25.9985, 0) construction
  line L17 (12.1998, -8.5) -> (-12.8827, -8.5) construction
  point P0 (0, 0)
  point P1 (11.55, -8.5)
  dimension "d530" = 4
  constraints: 26 point on line, 20 end point, 4 perpendicular, 2 horizontal, 1 midpoint, 3 other
  measures "d530" distance between parallel lines of L9 L8
extrude "Extrusion36" add sketch "Sketch10" along normal blind 3
fillet "Fillet3" radius 2 8 edges at (10.65, 5.5, -10.5) (10.65, 5.5, -6.5) (-10.65, 5.5, -10.5) (-10.65, 5.5, -6.5) (-10.65, 5.5, 6.5) (-10.65, 5.5, 10.5) (10.65, 5.5, 6.5) (10.65, 5.5, 10.5)
body "Solid4"
